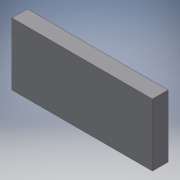
# Autodesk Inventor part: XcolBracket
Saved by Autodesk Inventor 2019 (Build 230136000, 136)
## iProperties
Created: 2018-10-03
Part Number: XcolBracket
Material: Aluminum 6061-AHC
Document SubType Name: Modeling
Designer: LillaHunden
Mass: 97.2 g
Surface Area: 98 cm^2
Volume: 36 cm^3
Density: 2.7 g/cm^3
Appearance: Aluminum - Dark
Author: LillaHunden
Autodesk Inventor part; units mm, degrees
ref_plane "YZ Plane" through (0, 0, 0) normal (1, 0, 0) x (0, 1, 0)
ref_plane "XZ Plane" through (0, 0, 0) normal (0, 1, 0) x (-1, 0, 0)
ref_plane "XY Plane" through (0, 0, 0) normal (0, 0, 1) x (1, 0, 0)
sketch "Sketch1" plane through (0, 0, 0) normal (0, 0, 1) x (1, 0, 0)
  line L0 (22.4756, 14.1051) -> (-67.5244, 14.1051)
  line L1 (-67.5244, 14.1051) -> (-67.5244, -25.8949)
  line L2 (-67.5244, -25.8949) -> (22.4756, -25.8949)
  line L3 (22.4756, -25.8949) -> (22.4756, 14.1051)
  point P0 (0, 0)
  dimension "d0" = 90
  dimension "d1" = 40
  constraints: 8 end point, 2 parallel, 1 horizontal, 1 perpendicular
  measures "d0" distance of L2.end L1.end
  measures "d1" distance of L1.end L0.end
extrude "Extrusion1" add sketch "Sketch1" along normal blind 10
body "Solid1"
